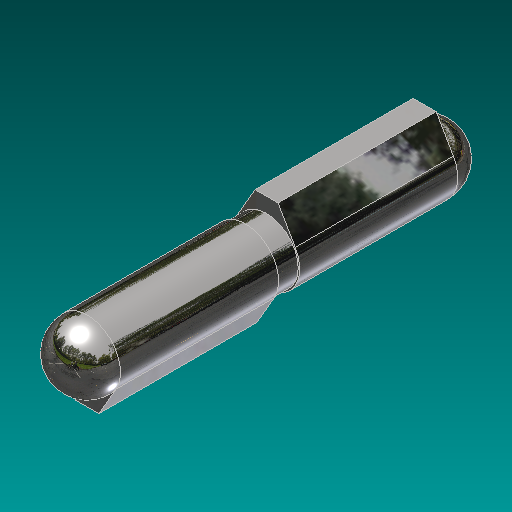
# Autodesk Inventor part: Weld-on hinge #218-109
Saved by Autodesk Inventor 2017 (Build 210142000, 142)
## iProperties
Created: 2013-06-12
Part Number: Weld-on hinge #218-109
Material: Stainless Steel
Document SubType Name: Modeling
Designer: Graeme_Van_Dongen
Density: 8.08 g/cm^3
Description: WELD-ON HINGE, STAINLESS, GREGG #218-109
Appearance: Semi-Polished
Mass: 40.8705 g
Surface Area: 21.288 cm^2
Volume: 5.05823 cm^3
Author: Graeme_Van_Dongen
Autodesk Inventor part; units mm, degrees
ref_plane "YZ Plane" through (0, 0, 0) normal (1, 0, 0) x (0, 1, 0)
ref_plane "XZ Plane" through (0, 0, 0) normal (0, 1, 0) x (-1, 0, 0)
ref_plane "XY Plane" through (0, 0, 0) normal (0, 0, 1) x (1, 0, 0)
sketch "Sketch1" plane through (0, 0, 0) normal (0, 0, 1) x (1, 0, 0)
  circle A0 centre (0, 0) radius 4.7625
  dimension "d0" = 9.525
  constraints: 1 centre point, 1 coincident
  measures "d0" diameter of A0
extrude "Extrusion1" add sketch "Sketch1" along normal mid plane 3.175
sketch "Sketch2" plane through (0, 0, 1.5875) normal (0, 0, 1) x (1, 0, 0)
  circle A0 centre (0, 0) radius 4.7625 construction
  line L0 (-1.7321, -7) -> (1.7321, -7)
  line L1 (1.7321, -7) -> (4.3301, -2.5)
  line L2 (-1.7321, -7) -> (-4.3301, -2.5)
  arc A1 (4.3301, -2.5) -> (-4.3301, -2.5) centre (0, 0) ccw
  dimension "d4" = 60
  dimension "d10" = 12
  dimension "d12" = 10
  constraints: 6 end point, 2 point on circle, 2 tangent, 1 centre point, 1 concentric, 1 equal length, 1 horizontal
  measures "d4" angle of L1 L2
  measures "d12" diameter of A1
extrude "Extrusion2" add sketch "Sketch2" along normal blind 23.8125
sketch "Sketch3" plane through (0, 0, -1.5875) normal (0, 0, -1) x (-1, 0, 0)
  circle A0 centre (0, 0) radius 4.7625 construction
  line L0 (4.3301, 2.5) -> (1.7321, 7)
  line L1 (1.7321, 7) -> (-1.7321, 7)
  line L2 (-1.7321, 7) -> (-4.3301, 2.5)
  arc A1 (-4.3301, 2.5) -> (4.3301, 2.5) centre (0, 0) ccw
  line L3 (4.3301, -2.5) -> (1.7321, -7) construction
  line L4 (1.7321, -7) -> (-1.7321, -7) construction
  dimension "d13" = 10
  constraints: 6 end point, 3 equal length, 2 point on circle, 2 tangent, 1 centre point, 1 concentric, 1 horizontal
  measures "d13" diameter of A1
extrude "Extrusion3" add sketch "Sketch3" along normal blind 23.8125
sketch "Sketch4" plane through (0, 0, 0) normal (1, 0, 0) x (0, 1, 0)
  line L0 (5, 25.4) -> (-2.5, 25.4) construction
  line L1 (-5, -25.4) -> (2.5, -25.4) construction
  line L2 (0, -44.0097) -> (0, 44.0097) construction
  line L3 (0, 25.4) -> (5, 25.4)
  line L4 (0, 25.4) -> (0, 30.4)
  arc A0 (5, 25.4) -> (0, 30.4) centre (0, 25.4) ccw
  line L5 (5, -25.4) -> (0, -25.4)
  line L6 (0, -25.4) -> (0, -30.4)
  arc A1 (0, -30.4) -> (5, -25.4) centre (0, -25.4) ccw
  point P0 (0, 0)
  constraints: 8 end point, 7 point on line, 4 point on circle, 3 equal length, 2 centre point, 2 line through centre, 1 collinear
revolve "Revolution1" add sketch "Sketch4" angle 360 about axis through (0, 0, -10) along (0, 0, 1)
equation "\"d7\" = d5"
equation "\"d5\" = 23.8125"
body "Solid1"
